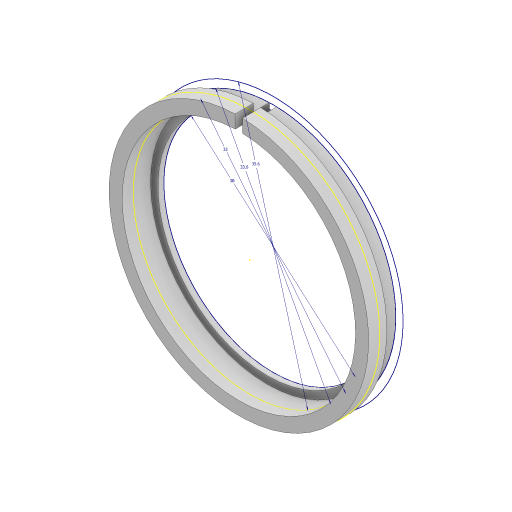
# Autodesk Inventor part: 32to36mm-FilterAdapter
Saved by Autodesk Inventor 2023 (Build 270158000, 158)
## iProperties
Created: 2022-11-22
Part Number: 32to36mm-FilterAdapter
Material: Generic
Document SubType Name: Modeling
Designer: nvladi
Density: 1 g/cm^3
Appearance: Default
Author: nvladi
Autodesk Inventor part; units mm, degrees
ref_plane "YZ Plane" through (0, 0, 0) normal (1, 0, 0) x (0, 1, 0)
ref_plane "XZ Plane" through (0, 0, 0) normal (0, 1, 0) x (-1, 0, 0)
ref_plane "XY Plane" through (0, 0, 0) normal (0, 0, 1) x (1, 0, 0)
sketch "Sketch1" plane through (0, 0, 0) normal (0, 0, 1) x (1, 0, 0)
  circle A0 centre (0, 0) radius 16.8
  circle A1 centre (0, 0) radius 15
  circle A2 centre (0, 0) radius 17.8
  circle A3 centre (0, 0) radius 16
  dimension "d0" = 33.6
  dimension "d1" = 30
  dimension "d2" = 35.6
  dimension "d3" = 32
  constraints: 4 centre point, 4 coincident
  measures "d0" diameter of A0
  measures "d1" diameter of A1
  measures "d2" diameter of A2
  measures "d3" diameter of A3
extrude "Extrusion1" add sketch "Sketch1" along normal blind 0.8 contours A3
extrude "Extrusion2" add sketch "Sketch1" along normal blind 3.2 contours A0
sketch "Sketch2" plane through (0, 0, 3.2) normal (0, 0, 1) x (1, 0, 0)
  circle A0 centre (0, 0) radius 17.8 projected
  circle A1 centre (0, 0) radius 16 projected
extrude "Extrusion3" add sketch "Sketch2" along normal blind 1.5
extrude "Extrusion5" add sketch "Sketch2" against normal blind 1
sketch "Sketch3" plane through (0, 0, 4.7) normal (0, 0, 1) x (1, 0, 0)
  line L0 (0.5, 8) -> (-0.5, 8)
  line L1 (-0.5, 8) -> (-0.5, 24)
  line L2 (-0.5, 24) -> (0.5, 24)
  line L3 (0.5, 24) -> (0.5, 8)
  circle A0 centre (0, 0) radius 16 projected
  line L4 (0.5, 8) -> (-0.5, 24) construction
  line L5 (-0.5, 8) -> (0.5, 24) construction
  point P0 (0, 16)
  dimension "d10" = 1
  dimension "d11" = 16
  constraints: 12 end point, 2 midpoint, 2 parallel, 1 horizontal, 1 perpendicular, 1 vertical alignment, 1 other
  measures "d10" distance of L1.end L2.end
  measures "d11" distance of L0.end L1.end
extrude "Extrusion4" cut sketch "Sketch3" against normal blind 10 contours L0 L1 A0 L3 | A0 L1 L2 L3 picked at (0.0556, 10.6664)
body "Solid1"
